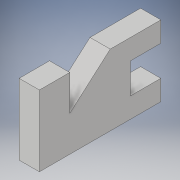
# Autodesk Inventor part: P2-1
Saved by Autodesk Inventor 2017 (Build 210142000, 142)
## iProperties
Created: 2017-02-09
Part Number: P2-1
Material: Generic
Document SubType Name: Modeling
Designer: Schaffel
Density: 1 g/cm^3
Appearance: Default
Author: Schaffel
Autodesk Inventor part; units mm, degrees
ref_plane "YZ Plane" through (0, 0, 0) normal (1, 0, 0) x (0, 1, 0)
ref_plane "XZ Plane" through (0, 0, 0) normal (0, 1, 0) x (-1, 0, 0)
ref_plane "XY Plane" through (0, 0, 0) normal (0, 0, 1) x (1, 0, 0)
sketch "Sketch1" plane through (0, 0, 0) normal (1, 0, 0) x (0, 1, 0)
  line L0 (0, 0) -> (0, -152.4)
  line L1 (0, -152.4) -> (25.4, -152.4)
  line L2 (25.4, -152.4) -> (25.4, -114.3)
  line L3 (25.4, -114.3) -> (63.5, -114.3)
  line L4 (63.5, -114.3) -> (63.5, -152.4)
  line L5 (63.5, -152.4) -> (88.9, -152.4)
  line L6 (88.9, -152.4) -> (88.9, -88.9)
  line L7 (0, 0) -> (88.9, 0)
  line L8 (88.9, 0) -> (88.9, -38.1)
  line L9 (88.9, -38.1) -> (44.45, -38.1)
  line L10 (44.45, -38.1) -> (88.9, -88.9)
  dimension "d0" = 152.4
  constraints: 22 end point, 7 perpendicular, 2 point on line, 1 horizontal, 1 vertical
  measures "d0" distance of L0.start L0.end
extrude "Extrusion1" add sketch "Sketch1" along normal blind 25.4
body "Solid1"
